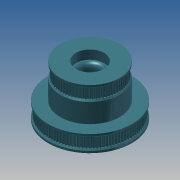
# Autodesk Inventor part: SCREW Z IDLER
Saved by Autodesk Inventor 2013 (Build 170138000, 138)
## iProperties
Created: 2017-04-04
Part Number: SCREW Z IDLER
Material: Generic
Document SubType Name: Modeling
Designer: employee
Density: 1 g/cm^3
Author: employee
Autodesk Inventor part; units mm, degrees
ref_plane "YZ Plane" through (0, 0, 0) normal (1, 0, 0) x (0, 1, 0)
ref_plane "XZ Plane" through (0, 0, 0) normal (0, 1, 0) x (-1, 0, 0)
ref_plane "XY Plane" through (0, 0, 0) normal (0, 0, 1) x (1, 0, 0)
sketch "Sketch1" plane through (0, 0, 0) normal (0, 0, 1) x (1, 0, 0)
  circle A0 centre (0, 0) radius 22.2817
  dimension "d0" = 44.5634
  constraints: 1 centre point, 1 coincident
  measures "d0" diameter of A0
extrude "Extrusion1" add sketch "Sketch1" along normal blind 8
sketch "Sketch2" plane through (0, 0, 8) normal (0, 0, 1) x (1, 0, 0)
  circle A0 centre (0, 0) radius 22.2817 projected
  circle A1 centre (0, 22.2817) radius 0.795
  dimension "d4" = 1.59
  constraints: 2 vertical alignment, 1 centre point, 1 other
  measures "d4" diameter of A1
extrude "Extrusion2" cut sketch "Sketch2" against normal through all contours A1 A0 | A0 A1 picked at (0.0316, 22.0175) picked at (0.0298, 22.544)
pattern_circular "Circular Pattern1" count 70 over 360 about axis through (0, 0, 0) along (0, 0, 1) of "Extrusion2"
sketch "Sketch3" plane through (0, 0, 8) normal (0, 0, 1) x (1, 0, 0)
  arc A0 (1.2044, 22.2491) -> (2.7877, 22.1066) centre (1.9973, 22.192) ccw projected
  arc A1 (1.2044, 22.2491) -> (0.7949, 22.2675) centre (0, 0) ccw projected
  arc A2 (-0.7949, 22.2675) -> (0.7949, 22.2675) centre (0, 22.2817) ccw projected
  arc A3 (-0.7949, 22.2675) -> (-1.2044, 22.2491) centre (0, 0) ccw projected
  arc A4 (-2.7877, 22.1066) -> (-1.2044, 22.2491) centre (-1.9973, 22.192) ccw projected
  arc A5 (-2.7877, 22.1066) -> (-3.1939, 22.0516) centre (0, 0) ccw projected
  arc A6 (-4.7581, 21.7677) -> (-3.1939, 22.0516) centre (-3.9785, 21.9236) ccw projected
  arc A7 (-4.7581, 21.7677) -> (-5.1577, 21.6765) centre (0, 0) ccw projected
  arc A8 (-6.6902, 21.2536) -> (-5.1577, 21.6765) centre (-5.9278, 21.4787) ccw projected
  arc A9 (-6.6902, 21.2536) -> (-7.0801, 21.1269) centre (0, 0) ccw projected
  arc A10 (-8.5684, 20.5683) -> (-7.0801, 21.1269) centre (-7.8292, 20.8609) ccw projected
  arc A11 (-8.5684, 20.5683) -> (-8.9454, 20.4072) centre (0, 0) ccw projected
  arc A12 (-10.3777, 19.7175) -> (-8.9454, 20.4072) centre (-9.6677, 20.0751) ccw projected
  arc A13 (-10.3777, 19.7175) -> (-10.7386, 19.5232) centre (0, 0) ccw projected
  arc A14 (-12.1033, 18.7078) -> (-10.7386, 19.5232) centre (-11.4283, 19.1277) ccw projected
  arc A15 (-12.1033, 18.7078) -> (-12.4454, 18.482) centre (0, 0) ccw projected
  arc A16 (-13.7316, 17.5476) -> (-12.4454, 18.482) centre (-13.0968, 18.0263) ccw projected
  arc A17 (-13.7316, 17.5476) -> (-14.0521, 17.292) centre (0, 0) ccw projected
  arc A18 (-15.2493, 16.246) -> (-14.0521, 17.292) centre (-14.66, 16.7797) ccw projected
  arc A19 (-15.2493, 16.246) -> (-15.5455, 15.9628) centre (0, 0) ccw projected
  arc A20 (-16.6441, 14.8137) -> (-15.5455, 15.9628) centre (-16.1051, 15.398) ccw projected
  arc A21 (-16.6441, 14.8137) -> (-16.9138, 14.505) centre (0, 0) ccw projected
  arc A22 (-17.905, 13.2621) -> (-16.9138, 14.505) centre (-17.4205, 13.8924) ccw projected
  arc A23 (-17.905, 13.2621) -> (-18.146, 12.9305) centre (0, 0) ccw projected
  arc A24 (-19.0218, 11.6037) -> (-18.146, 12.9305) centre (-18.5957, 12.2749) ccw projected
  arc A25 (-19.0218, 11.6037) -> (-19.232, 11.2518) centre (0, 0) ccw projected
  arc A26 (-19.9853, 9.8519) -> (-19.232, 11.2518) centre (-19.6212, 10.5586) ccw projected
  arc A27 (-19.9853, 9.8519) -> (-20.1632, 9.4826) centre (0, 0) ccw projected
  arc A28 (-20.788, 8.0208) -> (-20.1632, 9.4826) centre (-20.4886, 8.7573) ccw projected
  arc A29 (-20.788, 8.0208) -> (-20.932, 7.637) centre (0, 0) ccw projected
  arc A30 (-21.4233, 6.1251) -> (-20.932, 7.637) centre (-21.1911, 6.8854) ccw projected
  arc A31 (-21.4233, 6.1251) -> (-21.5323, 5.7299) centre (0, 0) ccw projected
  arc A32 (-21.8861, 4.18) -> (-21.5323, 5.7299) centre (-21.723, 4.9581) ccw projected
  arc A33 (-21.8861, 4.18) -> (-21.9593, 3.7767) centre (0, 0) ccw projected
  arc A34 (-22.1727, 2.2014) -> (-21.9593, 3.7767) centre (-22.08, 2.9909) ccw projected
  arc A35 (-22.1727, 2.2014) -> (-22.2094, 1.7931) centre (0, 0) ccw projected
  arc A36 (-22.2807, 0.205) -> (-22.2094, 1.7931) centre (-22.2593, 0.9997) ccw projected
  arc A37 (-22.2807, 0.205) -> (-22.2807, -0.205) centre (0, 0) ccw projected
  arc A38 (-22.2094, -1.7931) -> (-22.2807, -0.205) centre (-22.2593, -0.9997) ccw projected
  arc A39 (-22.2094, -1.7931) -> (-22.1727, -2.2014) centre (0, 0) ccw projected
  arc A40 (-21.9593, -3.7767) -> (-22.1727, -2.2014) centre (-22.08, -2.9909) ccw projected
  arc A41 (-21.9593, -3.7767) -> (-21.8861, -4.18) centre (0, 0) ccw projected
  arc A42 (-21.5323, -5.7299) -> (-21.8861, -4.18) centre (-21.723, -4.9581) ccw projected
  arc A43 (-21.5323, -5.7299) -> (-21.4233, -6.1251) centre (0, 0) ccw projected
  arc A44 (-20.932, -7.637) -> (-21.4233, -6.1251) centre (-21.1911, -6.8854) ccw projected
  arc A45 (-20.932, -7.637) -> (-20.788, -8.0208) centre (0, 0) ccw projected
  arc A46 (-20.1632, -9.4826) -> (-20.788, -8.0208) centre (-20.4886, -8.7573) ccw projected
  arc A47 (-20.1632, -9.4826) -> (-19.9853, -9.8519) centre (0, 0) ccw projected
  arc A48 (-19.232, -11.2518) -> (-19.9853, -9.8519) centre (-19.6212, -10.5586) ccw projected
  arc A49 (-19.232, -11.2518) -> (-19.0218, -11.6037) centre (0, 0) ccw projected
  arc A50 (-18.146, -12.9305) -> (-19.0218, -11.6037) centre (-18.5957, -12.2749) ccw projected
  arc A51 (-18.146, -12.9305) -> (-17.905, -13.2621) centre (0, 0) ccw projected
  arc A52 (-16.9138, -14.505) -> (-17.905, -13.2621) centre (-17.4205, -13.8924) ccw projected
  arc A53 (-16.9138, -14.505) -> (-16.6441, -14.8137) centre (0, 0) ccw projected
  arc A54 (-15.5455, -15.9628) -> (-16.6441, -14.8137) centre (-16.1051, -15.398) ccw projected
  arc A55 (-15.5455, -15.9628) -> (-15.2493, -16.246) centre (0, 0) ccw projected
  arc A56 (-14.0521, -17.292) -> (-15.2493, -16.246) centre (-14.66, -16.7797) ccw projected
  arc A57 (-14.0521, -17.292) -> (-13.7316, -17.5476) centre (0, 0) ccw projected
  arc A58 (-12.4454, -18.482) -> (-13.7316, -17.5476) centre (-13.0968, -18.0263) ccw projected
  arc A59 (-12.4454, -18.482) -> (-12.1033, -18.7078) centre (0, 0) ccw projected
  arc A60 (-10.7386, -19.5232) -> (-12.1033, -18.7078) centre (-11.4283, -19.1277) ccw projected
  arc A61 (-10.7386, -19.5232) -> (-10.3777, -19.7175) centre (0, 0) ccw projected
  arc A62 (-8.9454, -20.4072) -> (-10.3777, -19.7175) centre (-9.6677, -20.0751) ccw projected
  arc A63 (-8.9454, -20.4072) -> (-8.5684, -20.5683) centre (0, 0) ccw projected
  arc A64 (-7.0801, -21.1269) -> (-8.5684, -20.5683) centre (-7.8292, -20.8609) ccw projected
  arc A65 (-7.0801, -21.1269) -> (-6.6902, -21.2536) centre (0, 0) ccw projected
  arc A66 (-5.1577, -21.6765) -> (-6.6902, -21.2536) centre (-5.9278, -21.4787) ccw projected
  arc A67 (-5.1577, -21.6765) -> (-4.7581, -21.7677) centre (0, 0) ccw projected
  arc A68 (-3.1939, -22.0516) -> (-4.7581, -21.7677) centre (-3.9785, -21.9236) ccw projected
  arc A69 (-3.1939, -22.0516) -> (-2.7877, -22.1066) centre (0, 0) ccw projected
  arc A70 (-1.2044, -22.2491) -> (-2.7877, -22.1066) centre (-1.9973, -22.192) ccw projected
  arc A71 (-1.2044, -22.2491) -> (-0.7949, -22.2675) centre (0, 0) ccw projected
  arc A72 (0.7949, -22.2675) -> (-0.7949, -22.2675) centre (0, -22.2817) ccw projected
  arc A73 (0.7949, -22.2675) -> (1.2044, -22.2491) centre (0, 0) ccw projected
  arc A74 (2.7877, -22.1066) -> (1.2044, -22.2491) centre (1.9973, -22.192) ccw projected
  arc A75 (2.7877, -22.1066) -> (3.1939, -22.0516) centre (0, 0) ccw projected
  arc A76 (4.7581, -21.7677) -> (3.1939, -22.0516) centre (3.9785, -21.9236) ccw projected
  arc A77 (4.7581, -21.7677) -> (5.1577, -21.6765) centre (0, 0) ccw projected
  arc A78 (6.6902, -21.2536) -> (5.1577, -21.6765) centre (5.9278, -21.4787) ccw projected
  arc A79 (6.6902, -21.2536) -> (7.0801, -21.1269) centre (0, 0) ccw projected
  arc A80 (8.5684, -20.5683) -> (7.0801, -21.1269) centre (7.8292, -20.8609) ccw projected
  arc A81 (8.5684, -20.5683) -> (8.9454, -20.4072) centre (0, 0) ccw projected
  arc A82 (10.3777, -19.7175) -> (8.9454, -20.4072) centre (9.6677, -20.0751) ccw projected
  arc A83 (10.3777, -19.7175) -> (10.7386, -19.5232) centre (0, 0) ccw projected
  arc A84 (12.1033, -18.7078) -> (10.7386, -19.5232) centre (11.4283, -19.1277) ccw projected
  arc A85 (12.1033, -18.7078) -> (12.4454, -18.482) centre (0, 0) ccw projected
  arc A86 (13.7316, -17.5476) -> (12.4454, -18.482) centre (13.0968, -18.0263) ccw projected
  arc A87 (13.7316, -17.5476) -> (14.0521, -17.292) centre (0, 0) ccw projected
  arc A88 (15.2493, -16.246) -> (14.0521, -17.292) centre (14.66, -16.7797) ccw projected
  arc A89 (15.2493, -16.246) -> (15.5455, -15.9628) centre (0, 0) ccw projected
  arc A90 (16.6441, -14.8137) -> (15.5455, -15.9628) centre (16.1051, -15.398) ccw projected
  arc A91 (16.6441, -14.8137) -> (16.9138, -14.505) centre (0, 0) ccw projected
  arc A92 (17.905, -13.2621) -> (16.9138, -14.505) centre (17.4205, -13.8924) ccw projected
  arc A93 (17.905, -13.2621) -> (18.146, -12.9305) centre (0, 0) ccw projected
  arc A94 (19.0218, -11.6037) -> (18.146, -12.9305) centre (18.5957, -12.2749) ccw projected
  arc A95 (19.0218, -11.6037) -> (19.232, -11.2518) centre (0, 0) ccw projected
  arc A96 (19.9853, -9.8519) -> (19.232, -11.2518) centre (19.6212, -10.5586) ccw projected
  arc A97 (19.9853, -9.8519) -> (20.1632, -9.4826) centre (0, 0) ccw projected
  arc A98 (20.788, -8.0208) -> (20.1632, -9.4826) centre (20.4886, -8.7573) ccw projected
  arc A99 (20.788, -8.0208) -> (20.932, -7.637) centre (0, 0) ccw projected
  arc A100 (21.4233, -6.1251) -> (20.932, -7.637) centre (21.1911, -6.8854) ccw projected
  arc A101 (21.4233, -6.1251) -> (21.5323, -5.7299) centre (0, 0) ccw projected
  arc A102 (21.8861, -4.18) -> (21.5323, -5.7299) centre (21.723, -4.9581) ccw projected
  arc A103 (21.8861, -4.18) -> (21.9593, -3.7767) centre (0, 0) ccw projected
  arc A104 (22.1727, -2.2014) -> (21.9593, -3.7767) centre (22.08, -2.9909) ccw projected
  arc A105 (22.1727, -2.2014) -> (22.2094, -1.7931) centre (0, 0) ccw projected
  arc A106 (22.2807, -0.205) -> (22.2094, -1.7931) centre (22.2593, -0.9997) ccw projected
  arc A107 (22.2807, -0.205) -> (22.2807, 0.205) centre (0, 0) ccw projected
  arc A108 (22.2094, 1.7931) -> (22.2807, 0.205) centre (22.2593, 0.9997) ccw projected
  arc A109 (22.2094, 1.7931) -> (22.1727, 2.2014) centre (0, 0) ccw projected
  arc A110 (21.9593, 3.7767) -> (22.1727, 2.2014) centre (22.08, 2.9909) ccw projected
  arc A111 (21.9593, 3.7767) -> (21.8861, 4.18) centre (0, 0) ccw projected
  arc A112 (21.5323, 5.7299) -> (21.8861, 4.18) centre (21.723, 4.9581) ccw projected
  arc A113 (21.5323, 5.7299) -> (21.4233, 6.1251) centre (0, 0) ccw projected
  arc A114 (20.932, 7.637) -> (21.4233, 6.1251) centre (21.1911, 6.8854) ccw projected
  arc A115 (20.932, 7.637) -> (20.788, 8.0208) centre (0, 0) ccw projected
  arc A116 (20.1632, 9.4826) -> (20.788, 8.0208) centre (20.4886, 8.7573) ccw projected
  arc A117 (20.1632, 9.4826) -> (19.9853, 9.8519) centre (0, 0) ccw projected
  arc A118 (19.232, 11.2518) -> (19.9853, 9.8519) centre (19.6212, 10.5586) ccw projected
  arc A119 (19.232, 11.2518) -> (19.0218, 11.6037) centre (0, 0) ccw projected
  arc A120 (18.146, 12.9305) -> (19.0218, 11.6037) centre (18.5957, 12.2749) ccw projected
  arc A121 (18.146, 12.9305) -> (17.905, 13.2621) centre (0, 0) ccw projected
  arc A122 (16.9138, 14.505) -> (17.905, 13.2621) centre (17.4205, 13.8924) ccw projected
  arc A123 (16.9138, 14.505) -> (16.6441, 14.8137) centre (0, 0) ccw projected
  arc A124 (15.5455, 15.9628) -> (16.6441, 14.8137) centre (16.1051, 15.398) ccw projected
  arc A125 (15.5455, 15.9628) -> (15.2493, 16.246) centre (0, 0) ccw projected
  arc A126 (14.0521, 17.292) -> (15.2493, 16.246) centre (14.66, 16.7797) ccw projected
  arc A127 (14.0521, 17.292) -> (13.7316, 17.5476) centre (0, 0) ccw projected
  arc A128 (12.4454, 18.482) -> (13.7316, 17.5476) centre (13.0968, 18.0263) ccw projected
  arc A129 (12.4454, 18.482) -> (12.1033, 18.7078) centre (0, 0) ccw projected
  arc A130 (10.7386, 19.5232) -> (12.1033, 18.7078) centre (11.4283, 19.1277) ccw projected
  arc A131 (10.7386, 19.5232) -> (10.3777, 19.7175) centre (0, 0) ccw projected
  arc A132 (8.9454, 20.4072) -> (10.3777, 19.7175) centre (9.6677, 20.0751) ccw projected
  arc A133 (8.9454, 20.4072) -> (8.5684, 20.5683) centre (0, 0) ccw projected
  arc A134 (7.0801, 21.1269) -> (8.5684, 20.5683) centre (7.8292, 20.8609) ccw projected
  arc A135 (7.0801, 21.1269) -> (6.6902, 21.2536) centre (0, 0) ccw projected
  arc A136 (5.1577, 21.6765) -> (6.6902, 21.2536) centre (5.9278, 21.4787) ccw projected
  arc A137 (5.1577, 21.6765) -> (4.7581, 21.7677) centre (0, 0) ccw projected
  arc A138 (3.1939, 22.0516) -> (4.7581, 21.7677) centre (3.9785, 21.9236) ccw projected
  arc A139 (3.1939, 22.0516) -> (2.7877, 22.1066) centre (0, 0) ccw projected
  circle A140 centre (0, 0) radius 23.2817
  dimension "d11" = 1
  constraints: 1 centre point, 1 coincident
  measures "d11" radial gap between concentric circles of A35 A140
extrude "Extrusion3" add sketch "Sketch3" along normal blind 2.5 contours A0 A139 A138 A137 A136 A135 A134 A133 A132 A131 A130 A129 A128 A127 A126 A125 A124 A123 A122 A121 A120 A119 A118 A117 A116 A115 A114 A113 A112 A111 A110 A109 A108 A107 A106 A105 A104 A103 A102 A101 A100 A99 A98 A97 A96 A95 A94 A93 A92 A91 A90 A89 A88 A87 A86 A85 A84 A83 A82 A81 A80 A79 A78 A77 A76 A75 A74 A73 A72 A71 A70 A69 A68 A67 A66 A65 A64 A63 A62 A61 A60 A59 A58 A57 A56 A55 A54 A53 A52 A51 A50 A49 A48 A47 A46 A45 A44 A43 A42 A41 A40 A39 A38 A37 A36 A35 A34 A33 A32 A31 A30 A29 A28 A27 A26 A25 A24 A23 A22 A21 A20 A19 A18 A17 A16 A15 A14 A13 A12 A11 A10 A9 A8 A7 A6 A5 A4 A3 A2 A1 | A140
sketch "Sketch4" plane through (0, 0, 0) normal (0, 0, -1) x (-1, 0, 0)
  circle A0 centre (0, 0) radius 23.2817 projected
extrude "Extrusion4" add sketch "Sketch4" along normal blind 16.1
sketch "Sketch5" plane through (0, 0, -16.1) normal (0, 0, -1) x (-1, 0, 0)
  circle A0 centre (0, 0) radius 23.2817 projected
  circle A1 centre (0, 0) radius 31.831
  dimension "d16" = 63.662
  constraints: 1 centre point, 1 coincident
  measures "d16" diameter of A1
extrude "Extrusion5" add sketch "Sketch5" along normal blind 13 contours A0 | A1
sketch "Sketch6" plane through (0, 0, -29.1) normal (0, 0, -1) x (-1, 0, 0)
  circle A0 centre (0, 0) radius 31.831 projected
  circle A1 centre (0, 31.831) radius 0.795
  dimension "d20" = 1.59
  constraints: 2 vertical alignment, 1 centre point, 1 other
  measures "d20" diameter of A1
extrude "Extrusion6" cut sketch "Sketch6" against normal through all contours A1 A0 | A0 A1 picked at (-0.0317, 31.5672) picked at (0.0304, 32.0935)
pattern_circular "Circular Pattern2" count 100 over 360 about axis through (0, 0, -16.1) along (0, 0, -1) of "Extrusion6"
sketch "Sketch7" plane through (0, 0, -29.1) normal (0, 0, -1) x (-1, 0, 0)
  arc A0 (1.2047, 31.8082) -> (2.7914, 31.7084) centre (1.9987, 31.7682) ccw projected
  arc A1 (1.2047, 31.8082) -> (0.7949, 31.8211) centre (0, 0) ccw projected
  arc A2 (-0.7949, 31.8211) -> (0.7949, 31.8211) centre (0, 31.831) ccw projected
  arc A3 (-0.7949, 31.8211) -> (-1.2047, 31.8082) centre (0, 0) ccw projected
  arc A4 (-2.7914, 31.7084) -> (-1.2047, 31.8082) centre (-1.9987, 31.7682) ccw projected
  arc A5 (-2.7914, 31.7084) -> (-3.1996, 31.6698) centre (0, 0) ccw projected
  arc A6 (-4.7769, 31.4705) -> (-3.1996, 31.6698) centre (-3.9895, 31.58) ccw projected
  arc A7 (-4.7769, 31.4705) -> (-5.1818, 31.4064) centre (0, 0) ccw projected
  arc A8 (-6.7435, 31.1085) -> (-5.1818, 31.4064) centre (-5.9645, 31.2672) ccw projected
  arc A9 (-6.7435, 31.1085) -> (-7.1436, 31.019) centre (0, 0) ccw projected
  arc A10 (-8.6835, 30.6237) -> (-7.1436, 31.019) centre (-7.916, 30.831) ccw projected
  arc A11 (-8.6835, 30.6237) -> (-9.0772, 30.5093) centre (0, 0) ccw projected
  arc A12 (-10.5893, 30.018) -> (-9.0772, 30.5093) centre (-9.8363, 30.2731) ccw projected
  arc A13 (-10.5893, 30.018) -> (-10.975, 29.8791) centre (0, 0) ccw projected
  arc A14 (-12.4532, 29.2938) -> (-10.975, 29.8791) centre (-11.7178, 29.5957) ccw projected
  arc A15 (-12.4532, 29.2938) -> (-12.8295, 29.131) centre (0, 0) ccw projected
  arc A16 (-14.268, 28.4541) -> (-12.8295, 29.131) centre (-13.553, 28.8015) ccw projected
  arc A17 (-14.268, 28.4541) -> (-14.6333, 28.268) centre (0, 0) ccw projected
  arc A18 (-16.0265, 27.502) -> (-14.6333, 28.268) centre (-15.3347, 27.8937) ccw projected
  arc A19 (-16.0265, 27.502) -> (-16.3794, 27.2934) centre (0, 0) ccw projected
  arc A20 (-17.7218, 26.4415) -> (-16.3794, 27.2934) centre (-17.0559, 26.8758) ccw projected
  arc A21 (-17.7218, 26.4415) -> (-18.0608, 26.211) centre (0, 0) ccw projected
  arc A22 (-19.3471, 25.2765) -> (-18.0608, 26.211) centre (-18.7098, 25.7518) ccw projected
  arc A23 (-19.3471, 25.2765) -> (-19.671, 25.0253) centre (0, 0) ccw projected
  arc A24 (-20.896, 24.0118) -> (-19.671, 25.0253) centre (-20.2898, 24.5262) ccw projected
  arc A25 (-20.896, 24.0118) -> (-21.2035, 23.7407) centre (0, 0) ccw projected
  arc A26 (-22.3625, 22.6524) -> (-21.2035, 23.7407) centre (-21.7898, 23.2038) ccw projected
  arc A27 (-22.3625, 22.6524) -> (-22.6524, 22.3625) centre (0, 0) ccw projected
  arc A28 (-23.7407, 21.2035) -> (-22.6524, 22.3625) centre (-23.2038, 21.7898) ccw projected
  arc A29 (-23.7407, 21.2035) -> (-24.0118, 20.896) centre (0, 0) ccw projected
  arc A30 (-25.0253, 19.671) -> (-24.0118, 20.896) centre (-24.5262, 20.2898) ccw projected
  arc A31 (-25.0253, 19.671) -> (-25.2765, 19.3471) centre (0, 0) ccw projected
  arc A32 (-26.211, 18.0608) -> (-25.2765, 19.3471) centre (-25.7518, 18.7098) ccw projected
  arc A33 (-26.211, 18.0608) -> (-26.4415, 17.7218) centre (0, 0) ccw projected
  arc A34 (-27.2934, 16.3794) -> (-26.4415, 17.7218) centre (-26.8758, 17.0559) ccw projected
  arc A35 (-27.2934, 16.3794) -> (-27.502, 16.0265) centre (0, 0) ccw projected
  arc A36 (-28.268, 14.6333) -> (-27.502, 16.0265) centre (-27.8937, 15.3347) ccw projected
  arc A37 (-28.268, 14.6333) -> (-28.4541, 14.268) centre (0, 0) ccw projected
  arc A38 (-29.131, 12.8295) -> (-28.4541, 14.268) centre (-28.8015, 13.553) ccw projected
  arc A39 (-29.131, 12.8295) -> (-29.2938, 12.4532) centre (0, 0) ccw projected
  arc A40 (-29.8791, 10.975) -> (-29.2938, 12.4532) centre (-29.5957, 11.7178) ccw projected
  arc A41 (-29.8791, 10.975) -> (-30.018, 10.5893) centre (0, 0) ccw projected
  arc A42 (-30.5093, 9.0772) -> (-30.018, 10.5893) centre (-30.2731, 9.8363) ccw projected
  arc A43 (-30.5093, 9.0772) -> (-30.6237, 8.6835) centre (0, 0) ccw projected
  arc A44 (-31.019, 7.1436) -> (-30.6237, 8.6835) centre (-30.831, 7.916) ccw projected
  arc A45 (-31.019, 7.1436) -> (-31.1085, 6.7435) centre (0, 0) ccw projected
  arc A46 (-31.4064, 5.1818) -> (-31.1085, 6.7435) centre (-31.2672, 5.9645) ccw projected
  arc A47 (-31.4064, 5.1818) -> (-31.4705, 4.7769) centre (0, 0) ccw projected
  arc A48 (-31.6698, 3.1996) -> (-31.4705, 4.7769) centre (-31.58, 3.9895) ccw projected
  arc A49 (-31.6698, 3.1996) -> (-31.7084, 2.7914) centre (0, 0) ccw projected
  arc A50 (-31.8082, 1.2047) -> (-31.7084, 2.7914) centre (-31.7682, 1.9987) ccw projected
  arc A51 (-31.8082, 1.2047) -> (-31.8211, 0.7949) centre (0, 0) ccw projected
  arc A52 (-31.8211, -0.7949) -> (-31.8211, 0.7949) centre (-31.831, 0) ccw projected
  arc A53 (-31.8211, -0.7949) -> (-31.8082, -1.2047) centre (0, 0) ccw projected
  arc A54 (-31.7084, -2.7914) -> (-31.8082, -1.2047) centre (-31.7682, -1.9987) ccw projected
  arc A55 (-31.7084, -2.7914) -> (-31.6698, -3.1996) centre (0, 0) ccw projected
  arc A56 (-31.4705, -4.7769) -> (-31.6698, -3.1996) centre (-31.58, -3.9895) ccw projected
  arc A57 (-31.4705, -4.7769) -> (-31.4064, -5.1818) centre (0, 0) ccw projected
  arc A58 (-31.1085, -6.7435) -> (-31.4064, -5.1818) centre (-31.2672, -5.9645) ccw projected
  arc A59 (-31.1085, -6.7435) -> (-31.019, -7.1436) centre (0, 0) ccw projected
  arc A60 (-30.6237, -8.6835) -> (-31.019, -7.1436) centre (-30.831, -7.916) ccw projected
  arc A61 (-30.6237, -8.6835) -> (-30.5093, -9.0772) centre (0, 0) ccw projected
  arc A62 (-30.018, -10.5893) -> (-30.5093, -9.0772) centre (-30.2731, -9.8363) ccw projected
  arc A63 (-30.018, -10.5893) -> (-29.8791, -10.975) centre (0, 0) ccw projected
  arc A64 (-29.2938, -12.4532) -> (-29.8791, -10.975) centre (-29.5957, -11.7178) ccw projected
  arc A65 (-29.2938, -12.4532) -> (-29.131, -12.8295) centre (0, 0) ccw projected
  arc A66 (-28.4541, -14.268) -> (-29.131, -12.8295) centre (-28.8015, -13.553) ccw projected
  arc A67 (-28.4541, -14.268) -> (-28.268, -14.6333) centre (0, 0) ccw projected
  arc A68 (-27.502, -16.0265) -> (-28.268, -14.6333) centre (-27.8937, -15.3347) ccw projected
  arc A69 (-27.502, -16.0265) -> (-27.2934, -16.3794) centre (0, 0) ccw projected
  arc A70 (-26.4415, -17.7218) -> (-27.2934, -16.3794) centre (-26.8758, -17.0559) ccw projected
  arc A71 (-26.4415, -17.7218) -> (-26.211, -18.0608) centre (0, 0) ccw projected
  arc A72 (-25.2765, -19.3471) -> (-26.211, -18.0608) centre (-25.7518, -18.7098) ccw projected
  arc A73 (-25.2765, -19.3471) -> (-25.0253, -19.671) centre (0, 0) ccw projected
  arc A74 (-24.0118, -20.896) -> (-25.0253, -19.671) centre (-24.5262, -20.2898) ccw projected
  arc A75 (-24.0118, -20.896) -> (-23.7407, -21.2035) centre (0, 0) ccw projected
  arc A76 (-22.6524, -22.3625) -> (-23.7407, -21.2035) centre (-23.2038, -21.7898) ccw projected
  arc A77 (-22.6524, -22.3625) -> (-22.3625, -22.6524) centre (0, 0) ccw projected
  arc A78 (-21.2035, -23.7407) -> (-22.3625, -22.6524) centre (-21.7898, -23.2038) ccw projected
  arc A79 (-21.2035, -23.7407) -> (-20.896, -24.0118) centre (0, 0) ccw projected
  arc A80 (-19.671, -25.0253) -> (-20.896, -24.0118) centre (-20.2898, -24.5262) ccw projected
  arc A81 (-19.671, -25.0253) -> (-19.3471, -25.2765) centre (0, 0) ccw projected
  arc A82 (-18.0608, -26.211) -> (-19.3471, -25.2765) centre (-18.7098, -25.7518) ccw projected
  arc A83 (-18.0608, -26.211) -> (-17.7218, -26.4415) centre (0, 0) ccw projected
  arc A84 (-16.3794, -27.2934) -> (-17.7218, -26.4415) centre (-17.0559, -26.8758) ccw projected
  arc A85 (-16.3794, -27.2934) -> (-16.0265, -27.502) centre (0, 0) ccw projected
  arc A86 (-14.6333, -28.268) -> (-16.0265, -27.502) centre (-15.3347, -27.8937) ccw projected
  arc A87 (-14.6333, -28.268) -> (-14.268, -28.4541) centre (0, 0) ccw projected
  arc A88 (-12.8295, -29.131) -> (-14.268, -28.4541) centre (-13.553, -28.8015) ccw projected
  arc A89 (-12.8295, -29.131) -> (-12.4532, -29.2938) centre (0, 0) ccw projected
  arc A90 (-10.975, -29.8791) -> (-12.4532, -29.2938) centre (-11.7178, -29.5957) ccw projected
  arc A91 (-10.975, -29.8791) -> (-10.5893, -30.018) centre (0, 0) ccw projected
  arc A92 (-9.0772, -30.5093) -> (-10.5893, -30.018) centre (-9.8363, -30.2731) ccw projected
  arc A93 (-9.0772, -30.5093) -> (-8.6835, -30.6237) centre (0, 0) ccw projected
  arc A94 (-7.1436, -31.019) -> (-8.6835, -30.6237) centre (-7.916, -30.831) ccw projected
  arc A95 (-7.1436, -31.019) -> (-6.7435, -31.1085) centre (0, 0) ccw projected
  arc A96 (-5.1818, -31.4064) -> (-6.7435, -31.1085) centre (-5.9645, -31.2672) ccw projected
  arc A97 (-5.1818, -31.4064) -> (-4.7769, -31.4705) centre (0, 0) ccw projected
  arc A98 (-3.1996, -31.6698) -> (-4.7769, -31.4705) centre (-3.9895, -31.58) ccw projected
  arc A99 (-3.1996, -31.6698) -> (-2.7914, -31.7084) centre (0, 0) ccw projected
  arc A100 (-1.2047, -31.8082) -> (-2.7914, -31.7084) centre (-1.9987, -31.7682) ccw projected
  arc A101 (-1.2047, -31.8082) -> (-0.7949, -31.8211) centre (0, 0) ccw projected
  arc A102 (0.7949, -31.8211) -> (-0.7949, -31.8211) centre (0, -31.831) ccw projected
  arc A103 (0.7949, -31.8211) -> (1.2047, -31.8082) centre (0, 0) ccw projected
  arc A104 (2.7914, -31.7084) -> (1.2047, -31.8082) centre (1.9987, -31.7682) ccw projected
  arc A105 (2.7914, -31.7084) -> (3.1996, -31.6698) centre (0, 0) ccw projected
  arc A106 (4.7769, -31.4705) -> (3.1996, -31.6698) centre (3.9895, -31.58) ccw projected
  arc A107 (4.7769, -31.4705) -> (5.1818, -31.4064) centre (0, 0) ccw projected
  arc A108 (6.7435, -31.1085) -> (5.1818, -31.4064) centre (5.9645, -31.2672) ccw projected
  arc A109 (6.7435, -31.1085) -> (7.1436, -31.019) centre (0, 0) ccw projected
  arc A110 (8.6835, -30.6237) -> (7.1436, -31.019) centre (7.916, -30.831) ccw projected
  arc A111 (8.6835, -30.6237) -> (9.0772, -30.5093) centre (0, 0) ccw projected
  arc A112 (10.5893, -30.018) -> (9.0772, -30.5093) centre (9.8363, -30.2731) ccw projected
  arc A113 (10.5893, -30.018) -> (10.975, -29.8791) centre (0, 0) ccw projected
  arc A114 (12.4532, -29.2938) -> (10.975, -29.8791) centre (11.7178, -29.5957) ccw projected
  arc A115 (12.4532, -29.2938) -> (12.8295, -29.131) centre (0, 0) ccw projected
  arc A116 (14.268, -28.4541) -> (12.8295, -29.131) centre (13.553, -28.8015) ccw projected
  arc A117 (14.268, -28.4541) -> (14.6333, -28.268) centre (0, 0) ccw projected
  arc A118 (16.0265, -27.502) -> (14.6333, -28.268) centre (15.3347, -27.8937) ccw projected
  arc A119 (16.0265, -27.502) -> (16.3794, -27.2934) centre (0, 0) ccw projected
  arc A120 (17.7218, -26.4415) -> (16.3794, -27.2934) centre (17.0559, -26.8758) ccw projected
  arc A121 (17.7218, -26.4415) -> (18.0608, -26.211) centre (0, 0) ccw projected
  arc A122 (19.3471, -25.2765) -> (18.0608, -26.211) centre (18.7098, -25.7518) ccw projected
  arc A123 (19.3471, -25.2765) -> (19.671, -25.0253) centre (0, 0) ccw projected
  arc A124 (20.896, -24.0118) -> (19.671, -25.0253) centre (20.2898, -24.5262) ccw projected
  arc A125 (20.896, -24.0118) -> (21.2035, -23.7407) centre (0, 0) ccw projected
  arc A126 (22.3625, -22.6524) -> (21.2035, -23.7407) centre (21.7898, -23.2038) ccw projected
  arc A127 (22.3625, -22.6524) -> (22.6524, -22.3625) centre (0, 0) ccw projected
  arc A128 (23.7407, -21.2035) -> (22.6524, -22.3625) centre (23.2038, -21.7898) ccw projected
  arc A129 (23.7407, -21.2035) -> (24.0118, -20.896) centre (0, 0) ccw projected
  arc A130 (25.0253, -19.671) -> (24.0118, -20.896) centre (24.5262, -20.2898) ccw projected
  arc A131 (25.0253, -19.671) -> (25.2765, -19.3471) centre (0, 0) ccw projected
  arc A132 (26.211, -18.0608) -> (25.2765, -19.3471) centre (25.7518, -18.7098) ccw projected
  arc A133 (26.211, -18.0608) -> (26.4415, -17.7218) centre (0, 0) ccw projected
  arc A134 (27.2934, -16.3794) -> (26.4415, -17.7218) centre (26.8758, -17.0559) ccw projected
  arc A135 (27.2934, -16.3794) -> (27.502, -16.0265) centre (0, 0) ccw projected
  arc A136 (28.268, -14.6333) -> (27.502, -16.0265) centre (27.8937, -15.3347) ccw projected
  arc A137 (28.268, -14.6333) -> (28.4541, -14.268) centre (0, 0) ccw projected
  arc A138 (29.131, -12.8295) -> (28.4541, -14.268) centre (28.8015, -13.553) ccw projected
  arc A139 (29.131, -12.8295) -> (29.2938, -12.4532) centre (0, 0) ccw projected
  arc A140 (29.8791, -10.975) -> (29.2938, -12.4532) centre (29.5957, -11.7178) ccw projected
  arc A141 (29.8791, -10.975) -> (30.018, -10.5893) centre (0, 0) ccw projected
  arc A142 (30.5093, -9.0772) -> (30.018, -10.5893) centre (30.2731, -9.8363) ccw projected
  arc A143 (30.5093, -9.0772) -> (30.6237, -8.6835) centre (0, 0) ccw projected
  arc A144 (31.019, -7.1436) -> (30.6237, -8.6835) centre (30.831, -7.916) ccw projected
  arc A145 (31.019, -7.1436) -> (31.1085, -6.7435) centre (0, 0) ccw projected
  arc A146 (31.4064, -5.1818) -> (31.1085, -6.7435) centre (31.2672, -5.9645) ccw projected
  arc A147 (31.4064, -5.1818) -> (31.4705, -4.7769) centre (0, 0) ccw projected
  arc A148 (31.6698, -3.1996) -> (31.4705, -4.7769) centre (31.58, -3.9895) ccw projected
  arc A149 (31.6698, -3.1996) -> (31.7084, -2.7914) centre (0, 0) ccw projected
  arc A150 (31.8082, -1.2047) -> (31.7084, -2.7914) centre (31.7682, -1.9987) ccw projected
  arc A151 (31.8082, -1.2047) -> (31.8211, -0.7949) centre (0, 0) ccw projected
  arc A152 (31.8211, 0.7949) -> (31.8211, -0.7949) centre (31.831, 0) ccw projected
  arc A153 (31.8211, 0.7949) -> (31.8082, 1.2047) centre (0, 0) ccw projected
  arc A154 (31.7084, 2.7914) -> (31.8082, 1.2047) centre (31.7682, 1.9987) ccw projected
  arc A155 (31.7084, 2.7914) -> (31.6698, 3.1996) centre (0, 0) ccw projected
  arc A156 (31.4705, 4.7769) -> (31.6698, 3.1996) centre (31.58, 3.9895) ccw projected
  arc A157 (31.4705, 4.7769) -> (31.4064, 5.1818) centre (0, 0) ccw projected
  arc A158 (31.1085, 6.7435) -> (31.4064, 5.1818) centre (31.2672, 5.9645) ccw projected
  arc A159 (31.1085, 6.7435) -> (31.019, 7.1436) centre (0, 0) ccw projected
  arc A160 (30.6237, 8.6835) -> (31.019, 7.1436) centre (30.831, 7.916) ccw projected
  arc A161 (30.6237, 8.6835) -> (30.5093, 9.0772) centre (0, 0) ccw projected
  arc A162 (30.018, 10.5893) -> (30.5093, 9.0772) centre (30.2731, 9.8363) ccw projected
  arc A163 (30.018, 10.5893) -> (29.8791, 10.975) centre (0, 0) ccw projected
  arc A164 (29.2938, 12.4532) -> (29.8791, 10.975) centre (29.5957, 11.7178) ccw projected
  arc A165 (29.2938, 12.4532) -> (29.131, 12.8295) centre (0, 0) ccw projected
  arc A166 (28.4541, 14.268) -> (29.131, 12.8295) centre (28.8015, 13.553) ccw projected
  arc A167 (28.4541, 14.268) -> (28.268, 14.6333) centre (0, 0) ccw projected
  arc A168 (27.502, 16.0265) -> (28.268, 14.6333) centre (27.8937, 15.3347) ccw projected
  arc A169 (27.502, 16.0265) -> (27.2934, 16.3794) centre (0, 0) ccw projected
  arc A170 (26.4415, 17.7218) -> (27.2934, 16.3794) centre (26.8758, 17.0559) ccw projected
  arc A171 (26.4415, 17.7218) -> (26.211, 18.0608) centre (0, 0) ccw projected
  arc A172 (25.2765, 19.3471) -> (26.211, 18.0608) centre (25.7518, 18.7098) ccw projected
  arc A173 (25.2765, 19.3471) -> (25.0253, 19.671) centre (0, 0) ccw projected
  arc A174 (24.0118, 20.896) -> (25.0253, 19.671) centre (24.5262, 20.2898) ccw projected
  arc A175 (24.0118, 20.896) -> (23.7407, 21.2035) centre (0, 0) ccw projected
  arc A176 (22.6524, 22.3625) -> (23.7407, 21.2035) centre (23.2038, 21.7898) ccw projected
  arc A177 (22.6524, 22.3625) -> (22.3625, 22.6524) centre (0, 0) ccw projected
  arc A178 (21.2035, 23.7407) -> (22.3625, 22.6524) centre (21.7898, 23.2038) ccw projected
  arc A179 (21.2035, 23.7407) -> (20.896, 24.0118) centre (0, 0) ccw projected
  arc A180 (19.671, 25.0253) -> (20.896, 24.0118) centre (20.2898, 24.5262) ccw projected
  arc A181 (19.671, 25.0253) -> (19.3471, 25.2765) centre (0, 0) ccw projected
  arc A182 (18.0608, 26.211) -> (19.3471, 25.2765) centre (18.7098, 25.7518) ccw projected
  arc A183 (18.0608, 26.211) -> (17.7218, 26.4415) centre (0, 0) ccw projected
  arc A184 (16.3794, 27.2934) -> (17.7218, 26.4415) centre (17.0559, 26.8758) ccw projected
  arc A185 (16.3794, 27.2934) -> (16.0265, 27.502) centre (0, 0) ccw projected
  arc A186 (14.6333, 28.268) -> (16.0265, 27.502) centre (15.3347, 27.8937) ccw projected
  arc A187 (14.6333, 28.268) -> (14.268, 28.4541) centre (0, 0) ccw projected
  arc A188 (12.8295, 29.131) -> (14.268, 28.4541) centre (13.553, 28.8015) ccw projected
  arc A189 (12.8295, 29.131) -> (12.4532, 29.2938) centre (0, 0) ccw projected
  arc A190 (10.975, 29.8791) -> (12.4532, 29.2938) centre (11.7178, 29.5957) ccw projected
  arc A191 (10.975, 29.8791) -> (10.5893, 30.018) centre (0, 0) ccw projected
  arc A192 (9.0772, 30.5093) -> (10.5893, 30.018) centre (9.8363, 30.2731) ccw projected
  arc A193 (9.0772, 30.5093) -> (8.6835, 30.6237) centre (0, 0) ccw projected
  arc A194 (7.1436, 31.019) -> (8.6835, 30.6237) centre (7.916, 30.831) ccw projected
  arc A195 (7.1436, 31.019) -> (6.7435, 31.1085) centre (0, 0) ccw projected
  arc A196 (5.1818, 31.4064) -> (6.7435, 31.1085) centre (5.9645, 31.2672) ccw projected
  arc A197 (5.1818, 31.4064) -> (4.7769, 31.4705) centre (0, 0) ccw projected
  arc A198 (3.1996, 31.6698) -> (4.7769, 31.4705) centre (3.9895, 31.58) ccw projected
  arc A199 (3.1996, 31.6698) -> (2.7914, 31.7084) centre (0, 0) ccw projected
  circle A200 centre (0, 0) radius 32.831
  dimension "d27" = 1
  constraints: 1 centre point, 1 coincident
  measures "d27" radial gap between concentric circles of A51 A200
extrude "Extrusion7" add sketch "Sketch7" against normal blind 2.5
sketch "Sketch8" plane through (0, 0, -16.1) normal (0, 0, 1) x (1, 0, 0)
  arc A0 (-2.7914, 31.7084) -> (-1.2047, 31.8082) centre (-1.9987, 31.7682) ccw projected
  arc A1 (-2.7914, 31.7084) -> (-3.1996, 31.6698) centre (0, 0) ccw projected
  arc A2 (-4.7769, 31.4705) -> (-3.1996, 31.6698) centre (-3.9895, 31.58) ccw projected
  arc A3 (-4.7769, 31.4705) -> (-5.1818, 31.4064) centre (0, 0) ccw projected
  arc A4 (-6.7435, 31.1085) -> (-5.1818, 31.4064) centre (-5.9645, 31.2672) ccw projected
  arc A5 (-6.7435, 31.1085) -> (-7.1436, 31.019) centre (0, 0) ccw projected
  arc A6 (-8.6835, 30.6237) -> (-7.1436, 31.019) centre (-7.916, 30.831) ccw projected
  arc A7 (-8.6835, 30.6237) -> (-9.0772, 30.5093) centre (0, 0) ccw projected
  arc A8 (-10.5893, 30.018) -> (-9.0772, 30.5093) centre (-9.8363, 30.2731) ccw projected
  arc A9 (-10.5893, 30.018) -> (-10.975, 29.8791) centre (0, 0) ccw projected
  arc A10 (-12.4532, 29.2938) -> (-10.975, 29.8791) centre (-11.7178, 29.5957) ccw projected
  arc A11 (-12.4532, 29.2938) -> (-12.8295, 29.131) centre (0, 0) ccw projected
  arc A12 (-14.268, 28.4541) -> (-12.8295, 29.131) centre (-13.553, 28.8015) ccw projected
  arc A13 (-14.268, 28.4541) -> (-14.6333, 28.268) centre (0, 0) ccw projected
  arc A14 (-16.0265, 27.502) -> (-14.6333, 28.268) centre (-15.3347, 27.8937) ccw projected
  arc A15 (-16.0265, 27.502) -> (-16.3794, 27.2934) centre (0, 0) ccw projected
  arc A16 (-17.7218, 26.4415) -> (-16.3794, 27.2934) centre (-17.0559, 26.8758) ccw projected
  arc A17 (-17.7218, 26.4415) -> (-18.0608, 26.211) centre (0, 0) ccw projected
  arc A18 (-19.3471, 25.2765) -> (-18.0608, 26.211) centre (-18.7098, 25.7518) ccw projected
  arc A19 (-19.3471, 25.2765) -> (-19.671, 25.0253) centre (0, 0) ccw projected
  arc A20 (-20.896, 24.0118) -> (-19.671, 25.0253) centre (-20.2898, 24.5262) ccw projected
  arc A21 (-20.896, 24.0118) -> (-21.2035, 23.7407) centre (0, 0) ccw projected
  arc A22 (-22.3625, 22.6524) -> (-21.2035, 23.7407) centre (-21.7898, 23.2038) ccw projected
  arc A23 (-22.3625, 22.6524) -> (-22.6524, 22.3625) centre (0, 0) ccw projected
  arc A24 (-23.7407, 21.2035) -> (-22.6524, 22.3625) centre (-23.2038, 21.7898) ccw projected
  arc A25 (-23.7407, 21.2035) -> (-24.0118, 20.896) centre (0, 0) ccw projected
  arc A26 (-25.0253, 19.671) -> (-24.0118, 20.896) centre (-24.5262, 20.2898) ccw projected
  arc A27 (-25.0253, 19.671) -> (-25.2765, 19.3471) centre (0, 0) ccw projected
  arc A28 (-26.211, 18.0608) -> (-25.2765, 19.3471) centre (-25.7518, 18.7098) ccw projected
  arc A29 (-26.211, 18.0608) -> (-26.4415, 17.7218) centre (0, 0) ccw projected
  arc A30 (-27.2934, 16.3794) -> (-26.4415, 17.7218) centre (-26.8758, 17.0559) ccw projected
  arc A31 (-27.2934, 16.3794) -> (-27.502, 16.0265) centre (0, 0) ccw projected
  arc A32 (-28.268, 14.6333) -> (-27.502, 16.0265) centre (-27.8937, 15.3347) ccw projected
  arc A33 (-28.268, 14.6333) -> (-28.4541, 14.268) centre (0, 0) ccw projected
  arc A34 (-29.131, 12.8295) -> (-28.4541, 14.268) centre (-28.8015, 13.553) ccw projected
  arc A35 (-29.131, 12.8295) -> (-29.2938, 12.4532) centre (0, 0) ccw projected
  arc A36 (-29.8791, 10.975) -> (-29.2938, 12.4532) centre (-29.5957, 11.7178) ccw projected
  arc A37 (-29.8791, 10.975) -> (-30.018, 10.5893) centre (0, 0) ccw projected
  arc A38 (-30.5093, 9.0772) -> (-30.018, 10.5893) centre (-30.2731, 9.8363) ccw projected
  arc A39 (-30.5093, 9.0772) -> (-30.6237, 8.6835) centre (0, 0) ccw projected
  arc A40 (-31.019, 7.1436) -> (-30.6237, 8.6835) centre (-30.831, 7.916) ccw projected
  arc A41 (-31.019, 7.1436) -> (-31.1085, 6.7435) centre (0, 0) ccw projected
  arc A42 (-31.4064, 5.1818) -> (-31.1085, 6.7435) centre (-31.2672, 5.9645) ccw projected
  arc A43 (-31.4064, 5.1818) -> (-31.4705, 4.7769) centre (0, 0) ccw projected
  arc A44 (-31.6698, 3.1996) -> (-31.4705, 4.7769) centre (-31.58, 3.9895) ccw projected
  arc A45 (-31.6698, 3.1996) -> (-31.7084, 2.7914) centre (0, 0) ccw projected
  arc A46 (-31.8082, 1.2047) -> (-31.7084, 2.7914) centre (-31.7682, 1.9987) ccw projected
  arc A47 (-31.8082, 1.2047) -> (-31.8211, 0.7949) centre (0, 0) ccw projected
  arc A48 (-31.8211, -0.7949) -> (-31.8211, 0.7949) centre (-31.831, 0) ccw projected
  arc A49 (-31.8211, -0.7949) -> (-31.8082, -1.2047) centre (0, 0) ccw projected
  arc A50 (-31.7084, -2.7914) -> (-31.8082, -1.2047) centre (-31.7682, -1.9987) ccw projected
  arc A51 (-31.7084, -2.7914) -> (-31.6698, -3.1996) centre (0, 0) ccw projected
  arc A52 (-31.4705, -4.7769) -> (-31.6698, -3.1996) centre (-31.58, -3.9895) ccw projected
  arc A53 (-31.4705, -4.7769) -> (-31.4064, -5.1818) centre (0, 0) ccw projected
  arc A54 (-31.1085, -6.7435) -> (-31.4064, -5.1818) centre (-31.2672, -5.9645) ccw projected
  arc A55 (-31.1085, -6.7435) -> (-31.019, -7.1436) centre (0, 0) ccw projected
  arc A56 (-30.6237, -8.6835) -> (-31.019, -7.1436) centre (-30.831, -7.916) ccw projected
  arc A57 (-30.6237, -8.6835) -> (-30.5093, -9.0772) centre (0, 0) ccw projected
  arc A58 (-30.018, -10.5893) -> (-30.5093, -9.0772) centre (-30.2731, -9.8363) ccw projected
  arc A59 (-30.018, -10.5893) -> (-29.8791, -10.975) centre (0, 0) ccw projected
  arc A60 (-29.2938, -12.4532) -> (-29.8791, -10.975) centre (-29.5957, -11.7178) ccw projected
  arc A61 (-29.2938, -12.4532) -> (-29.131, -12.8295) centre (0, 0) ccw projected
  arc A62 (-28.4541, -14.268) -> (-29.131, -12.8295) centre (-28.8015, -13.553) ccw projected
  arc A63 (-28.4541, -14.268) -> (-28.268, -14.6333) centre (0, 0) ccw projected
  arc A64 (-27.502, -16.0265) -> (-28.268, -14.6333) centre (-27.8937, -15.3347) ccw projected
  arc A65 (-27.502, -16.0265) -> (-27.2934, -16.3794) centre (0, 0) ccw projected
  arc A66 (-26.4415, -17.7218) -> (-27.2934, -16.3794) centre (-26.8758, -17.0559) ccw projected
  arc A67 (-26.4415, -17.7218) -> (-26.211, -18.0608) centre (0, 0) ccw projected
  arc A68 (-25.2765, -19.3471) -> (-26.211, -18.0608) centre (-25.7518, -18.7098) ccw projected
  arc A69 (-25.2765, -19.3471) -> (-25.0253, -19.671) centre (0, 0) ccw projected
  arc A70 (-24.0118, -20.896) -> (-25.0253, -19.671) centre (-24.5262, -20.2898) ccw projected
  arc A71 (-24.0118, -20.896) -> (-23.7407, -21.2035) centre (0, 0) ccw projected
  arc A72 (-22.6524, -22.3625) -> (-23.7407, -21.2035) centre (-23.2038, -21.7898) ccw projected
  arc A73 (-22.6524, -22.3625) -> (-22.3625, -22.6524) centre (0, 0) ccw projected
  arc A74 (-21.2035, -23.7407) -> (-22.3625, -22.6524) centre (-21.7898, -23.2038) ccw projected
  arc A75 (-21.2035, -23.7407) -> (-20.896, -24.0118) centre (0, 0) ccw projected
  arc A76 (-19.671, -25.0253) -> (-20.896, -24.0118) centre (-20.2898, -24.5262) ccw projected
  arc A77 (-19.671, -25.0253) -> (-19.3471, -25.2765) centre (0, 0) ccw projected
  arc A78 (-18.0608, -26.211) -> (-19.3471, -25.2765) centre (-18.7098, -25.7518) ccw projected
  arc A79 (-18.0608, -26.211) -> (-17.7218, -26.4415) centre (0, 0) ccw projected
  arc A80 (-16.3794, -27.2934) -> (-17.7218, -26.4415) centre (-17.0559, -26.8758) ccw projected
  arc A81 (-16.3794, -27.2934) -> (-16.0265, -27.502) centre (0, 0) ccw projected
  arc A82 (-14.6333, -28.268) -> (-16.0265, -27.502) centre (-15.3347, -27.8937) ccw projected
  arc A83 (-14.6333, -28.268) -> (-14.268, -28.4541) centre (0, 0) ccw projected
  arc A84 (-12.8295, -29.131) -> (-14.268, -28.4541) centre (-13.553, -28.8015) ccw projected
  arc A85 (-12.8295, -29.131) -> (-12.4532, -29.2938) centre (0, 0) ccw projected
  arc A86 (-10.975, -29.8791) -> (-12.4532, -29.2938) centre (-11.7178, -29.5957) ccw projected
  arc A87 (-10.975, -29.8791) -> (-10.5893, -30.018) centre (0, 0) ccw projected
  arc A88 (-9.0772, -30.5093) -> (-10.5893, -30.018) centre (-9.8363, -30.2731) ccw projected
  arc A89 (-9.0772, -30.5093) -> (-8.6835, -30.6237) centre (0, 0) ccw projected
  arc A90 (-7.1436, -31.019) -> (-8.6835, -30.6237) centre (-7.916, -30.831) ccw projected
  arc A91 (-7.1436, -31.019) -> (-6.7435, -31.1085) centre (0, 0) ccw projected
  arc A92 (-5.1818, -31.4064) -> (-6.7435, -31.1085) centre (-5.9645, -31.2672) ccw projected
  arc A93 (-5.1818, -31.4064) -> (-4.7769, -31.4705) centre (0, 0) ccw projected
  arc A94 (-3.1996, -31.6698) -> (-4.7769, -31.4705) centre (-3.9895, -31.58) ccw projected
  arc A95 (-3.1996, -31.6698) -> (-2.7914, -31.7084) centre (0, 0) ccw projected
  arc A96 (-1.2047, -31.8082) -> (-2.7914, -31.7084) centre (-1.9987, -31.7682) ccw projected
  arc A97 (-1.2047, -31.8082) -> (-0.7949, -31.8211) centre (0, 0) ccw projected
  arc A98 (0.7949, -31.8211) -> (-0.7949, -31.8211) centre (0, -31.831) ccw projected
  arc A99 (0.7949, -31.8211) -> (1.2047, -31.8082) centre (0, 0) ccw projected
  arc A100 (2.7914, -31.7084) -> (1.2047, -31.8082) centre (1.9987, -31.7682) ccw projected
  arc A101 (2.7914, -31.7084) -> (3.1996, -31.6698) centre (0, 0) ccw projected
  arc A102 (4.7769, -31.4705) -> (3.1996, -31.6698) centre (3.9895, -31.58) ccw projected
  arc A103 (4.7769, -31.4705) -> (5.1818, -31.4064) centre (0, 0) ccw projected
  arc A104 (6.7435, -31.1085) -> (5.1818, -31.4064) centre (5.9645, -31.2672) ccw projected
  arc A105 (6.7435, -31.1085) -> (7.1436, -31.019) centre (0, 0) ccw projected
  arc A106 (8.6835, -30.6237) -> (7.1436, -31.019) centre (7.916, -30.831) ccw projected
  arc A107 (8.6835, -30.6237) -> (9.0772, -30.5093) centre (0, 0) ccw projected
  arc A108 (10.5893, -30.018) -> (9.0772, -30.5093) centre (9.8363, -30.2731) ccw projected
  arc A109 (10.5893, -30.018) -> (10.975, -29.8791) centre (0, 0) ccw projected
  arc A110 (12.4532, -29.2938) -> (10.975, -29.8791) centre (11.7178, -29.5957) ccw projected
  arc A111 (12.4532, -29.2938) -> (12.8295, -29.131) centre (0, 0) ccw projected
  arc A112 (14.268, -28.4541) -> (12.8295, -29.131) centre (13.553, -28.8015) ccw projected
  arc A113 (14.268, -28.4541) -> (14.6333, -28.268) centre (0, 0) ccw projected
  arc A114 (16.0265, -27.502) -> (14.6333, -28.268) centre (15.3347, -27.8937) ccw projected
  arc A115 (16.0265, -27.502) -> (16.3794, -27.2934) centre (0, 0) ccw projected
  arc A116 (17.7218, -26.4415) -> (16.3794, -27.2934) centre (17.0559, -26.8758) ccw projected
  arc A117 (17.7218, -26.4415) -> (18.0608, -26.211) centre (0, 0) ccw projected
  arc A118 (19.3471, -25.2765) -> (18.0608, -26.211) centre (18.7098, -25.7518) ccw projected
  arc A119 (19.3471, -25.2765) -> (19.671, -25.0253) centre (0, 0) ccw projected
  arc A120 (20.896, -24.0118) -> (19.671, -25.0253) centre (20.2898, -24.5262) ccw projected
  arc A121 (20.896, -24.0118) -> (21.2035, -23.7407) centre (0, 0) ccw projected
  arc A122 (22.3625, -22.6524) -> (21.2035, -23.7407) centre (21.7898, -23.2038) ccw projected
  arc A123 (22.3625, -22.6524) -> (22.6524, -22.3625) centre (0, 0) ccw projected
  arc A124 (23.7407, -21.2035) -> (22.6524, -22.3625) centre (23.2038, -21.7898) ccw projected
  arc A125 (23.7407, -21.2035) -> (24.0118, -20.896) centre (0, 0) ccw projected
  arc A126 (25.0253, -19.671) -> (24.0118, -20.896) centre (24.5262, -20.2898) ccw projected
  arc A127 (25.0253, -19.671) -> (25.2765, -19.3471) centre (0, 0) ccw projected
  arc A128 (26.211, -18.0608) -> (25.2765, -19.3471) centre (25.7518, -18.7098) ccw projected
  arc A129 (26.211, -18.0608) -> (26.4415, -17.7218) centre (0, 0) ccw projected
  arc A130 (27.2934, -16.3794) -> (26.4415, -17.7218) centre (26.8758, -17.0559) ccw projected
  arc A131 (27.2934, -16.3794) -> (27.502, -16.0265) centre (0, 0) ccw projected
  arc A132 (28.268, -14.6333) -> (27.502, -16.0265) centre (27.8937, -15.3347) ccw projected
  arc A133 (28.268, -14.6333) -> (28.4541, -14.268) centre (0, 0) ccw projected
  arc A134 (29.131, -12.8295) -> (28.4541, -14.268) centre (28.8015, -13.553) ccw projected
  arc A135 (29.131, -12.8295) -> (29.2938, -12.4532) centre (0, 0) ccw projected
  arc A136 (29.8791, -10.975) -> (29.2938, -12.4532) centre (29.5957, -11.7178) ccw projected
  arc A137 (29.8791, -10.975) -> (30.018, -10.5893) centre (0, 0) ccw projected
  arc A138 (30.5093, -9.0772) -> (30.018, -10.5893) centre (30.2731, -9.8363) ccw projected
  arc A139 (30.5093, -9.0772) -> (30.6237, -8.6835) centre (0, 0) ccw projected
  arc A140 (31.019, -7.1436) -> (30.6237, -8.6835) centre (30.831, -7.916) ccw projected
  arc A141 (31.019, -7.1436) -> (31.1085, -6.7435) centre (0, 0) ccw projected
  arc A142 (31.4064, -5.1818) -> (31.1085, -6.7435) centre (31.2672, -5.9645) ccw projected
  arc A143 (31.4064, -5.1818) -> (31.4705, -4.7769) centre (0, 0) ccw projected
  arc A144 (31.6698, -3.1996) -> (31.4705, -4.7769) centre (31.58, -3.9895) ccw projected
  arc A145 (31.6698, -3.1996) -> (31.7084, -2.7914) centre (0, 0) ccw projected
  arc A146 (31.8082, -1.2047) -> (31.7084, -2.7914) centre (31.7682, -1.9987) ccw projected
  arc A147 (31.8082, -1.2047) -> (31.8211, -0.7949) centre (0, 0) ccw projected
  arc A148 (31.8211, 0.7949) -> (31.8211, -0.7949) centre (31.831, 0) ccw projected
  arc A149 (31.8211, 0.7949) -> (31.8082, 1.2047) centre (0, 0) ccw projected
  arc A150 (31.7084, 2.7914) -> (31.8082, 1.2047) centre (31.7682, 1.9987) ccw projected
  arc A151 (31.7084, 2.7914) -> (31.6698, 3.1996) centre (0, 0) ccw projected
  arc A152 (31.4705, 4.7769) -> (31.6698, 3.1996) centre (31.58, 3.9895) ccw projected
  arc A153 (31.4705, 4.7769) -> (31.4064, 5.1818) centre (0, 0) ccw projected
  arc A154 (31.1085, 6.7435) -> (31.4064, 5.1818) centre (31.2672, 5.9645) ccw projected
  arc A155 (31.1085, 6.7435) -> (31.019, 7.1436) centre (0, 0) ccw projected
  arc A156 (30.6237, 8.6835) -> (31.019, 7.1436) centre (30.831, 7.916) ccw projected
  arc A157 (30.6237, 8.6835) -> (30.5093, 9.0772) centre (0, 0) ccw projected
  arc A158 (30.018, 10.5893) -> (30.5093, 9.0772) centre (30.2731, 9.8363) ccw projected
  arc A159 (30.018, 10.5893) -> (29.8791, 10.975) centre (0, 0) ccw projected
  arc A160 (29.2938, 12.4532) -> (29.8791, 10.975) centre (29.5957, 11.7178) ccw projected
  arc A161 (29.2938, 12.4532) -> (29.131, 12.8295) centre (0, 0) ccw projected
  arc A162 (28.4541, 14.268) -> (29.131, 12.8295) centre (28.8015, 13.553) ccw projected
  arc A163 (28.4541, 14.268) -> (28.268, 14.6333) centre (0, 0) ccw projected
  arc A164 (27.502, 16.0265) -> (28.268, 14.6333) centre (27.8937, 15.3347) ccw projected
  arc A165 (27.502, 16.0265) -> (27.2934, 16.3794) centre (0, 0) ccw projected
  arc A166 (26.4415, 17.7218) -> (27.2934, 16.3794) centre (26.8758, 17.0559) ccw projected
  arc A167 (26.4415, 17.7218) -> (26.211, 18.0608) centre (0, 0) ccw projected
  arc A168 (25.2765, 19.3471) -> (26.211, 18.0608) centre (25.7518, 18.7098) ccw projected
  arc A169 (25.2765, 19.3471) -> (25.0253, 19.671) centre (0, 0) ccw projected
  arc A170 (24.0118, 20.896) -> (25.0253, 19.671) centre (24.5262, 20.2898) ccw projected
  arc A171 (24.0118, 20.896) -> (23.7407, 21.2035) centre (0, 0) ccw projected
  arc A172 (22.6524, 22.3625) -> (23.7407, 21.2035) centre (23.2038, 21.7898) ccw projected
  arc A173 (22.6524, 22.3625) -> (22.3625, 22.6524) centre (0, 0) ccw projected
  arc A174 (21.2035, 23.7407) -> (22.3625, 22.6524) centre (21.7898, 23.2038) ccw projected
  arc A175 (21.2035, 23.7407) -> (20.896, 24.0118) centre (0, 0) ccw projected
  arc A176 (19.671, 25.0253) -> (20.896, 24.0118) centre (20.2898, 24.5262) ccw projected
  arc A177 (19.671, 25.0253) -> (19.3471, 25.2765) centre (0, 0) ccw projected
  arc A178 (18.0608, 26.211) -> (19.3471, 25.2765) centre (18.7098, 25.7518) ccw projected
  arc A179 (18.0608, 26.211) -> (17.7218, 26.4415) centre (0, 0) ccw projected
  arc A180 (16.3794, 27.2934) -> (17.7218, 26.4415) centre (17.0559, 26.8758) ccw projected
  arc A181 (16.3794, 27.2934) -> (16.0265, 27.502) centre (0, 0) ccw projected
  arc A182 (14.6333, 28.268) -> (16.0265, 27.502) centre (15.3347, 27.8937) ccw projected
  arc A183 (14.6333, 28.268) -> (14.268, 28.4541) centre (0, 0) ccw projected
  arc A184 (12.8295, 29.131) -> (14.268, 28.4541) centre (13.553, 28.8015) ccw projected
  arc A185 (12.8295, 29.131) -> (12.4532, 29.2938) centre (0, 0) ccw projected
  arc A186 (10.975, 29.8791) -> (12.4532, 29.2938) centre (11.7178, 29.5957) ccw projected
  arc A187 (10.975, 29.8791) -> (10.5893, 30.018) centre (0, 0) ccw projected
  arc A188 (9.0772, 30.5093) -> (10.5893, 30.018) centre (9.8363, 30.2731) ccw projected
  arc A189 (9.0772, 30.5093) -> (8.6835, 30.6237) centre (0, 0) ccw projected
  arc A190 (7.1436, 31.019) -> (8.6835, 30.6237) centre (7.916, 30.831) ccw projected
  arc A191 (7.1436, 31.019) -> (6.7435, 31.1085) centre (0, 0) ccw projected
  arc A192 (5.1818, 31.4064) -> (6.7435, 31.1085) centre (5.9645, 31.2672) ccw projected
  arc A193 (5.1818, 31.4064) -> (4.7769, 31.4705) centre (0, 0) ccw projected
  arc A194 (3.1996, 31.6698) -> (4.7769, 31.4705) centre (3.9895, 31.58) ccw projected
  arc A195 (3.1996, 31.6698) -> (2.7914, 31.7084) centre (0, 0) ccw projected
  arc A196 (1.2047, 31.8082) -> (2.7914, 31.7084) centre (1.9987, 31.7682) ccw projected
  arc A197 (1.2047, 31.8082) -> (0.7949, 31.8211) centre (0, 0) ccw projected
  arc A198 (-0.7949, 31.8211) -> (0.7949, 31.8211) centre (0, 31.831) ccw projected
  arc A199 (-0.7949, 31.8211) -> (-1.2047, 31.8082) centre (0, 0) ccw projected
  circle A200 centre (0, 0) radius 32.831 projected
extrude "Extrusion8" add sketch "Sketch8" against normal blind 2.5
chamfer "Chamfer1" distance 1 angle 45 4 edges at (32.831, 0, -26.6) (-32.831, 0, -18.6) (23.2817, 0, 0) (-23.2817, 0, 8)
sketch "Sketch9" plane through (0, 0, 10.5) normal (0, 0, 1) x (1, 0, 0)
  circle A0 centre (0, 0) radius 23.2817 projected
  circle A1 centre (0, 0) radius 7.5
  dimension "d35" = 15
  constraints: 1 centre point, 1 coincident
  measures "d35" diameter of A1
extrude "Extrusion9" cut sketch "Sketch9" against normal through all contours A1
sketch "Sketch10" plane through (0, 0, 10.5) normal (0, 0, 1) x (1, 0, 0)
  circle A0 centre (0, 0) radius 7.5 projected
  circle A1 centre (0, 0) radius 23.2817 projected
  circle A2 centre (0, 0) radius 11
  dimension "d39" = 22
  constraints: 1 centre point, 1 coincident
  measures "d39" diameter of A2
extrude "Extrusion10" cut sketch "Sketch10" against normal blind 7 contours A2
sketch "Sketch11" plane through (0, 0, -29.1) normal (0, 0, -1) x (-1, 0, 0)
  circle A0 centre (0, 0) radius 7.5 projected
  circle A1 centre (0, 0) radius 11 projected
extrude "Extrusion11" cut sketch "Sketch11" against normal blind 7
fillet "Fillet1" radius 3.5 2 edges at (-7.5, 0, -22.1) (-7.5, 0, 3.5)
body "Solid1"
